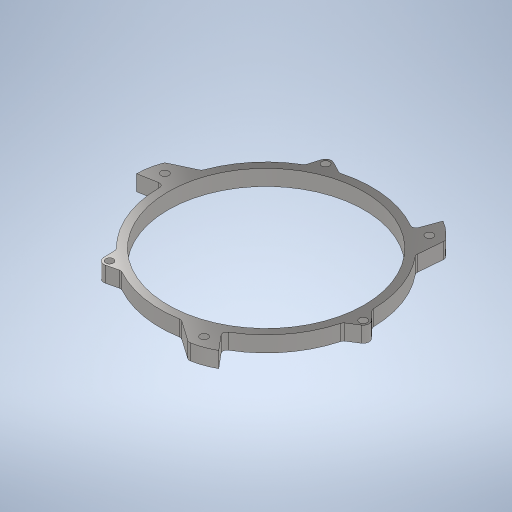
# Autodesk Inventor part: Blade V2
Saved by Autodesk Inventor 2023.2 (Build 272271000, 271)
## iProperties
Created: 2022-12-02
Part Number: Blade V2
Material: Stainless Steel
Document SubType Name: Modeling
Designer: Nathan Cai
Density: 8 g/cm^3
Appearance: Semi-Polished
Mass: 462.442 g
Surface Area: 248.364 cm^2
Volume: 57.8053 cm^3
Ring_ID: 6.250 in
ToothDepth: 0.750 in
RingWD: 0.250 in
Author: Nathan Cai
Autodesk Inventor part; units mm, degrees
ref_plane "YZ Plane" through (0, 0, 0) normal (1, 0, 0) x (0, 1, 0)
ref_plane "XZ Plane" through (0, 0, 0) normal (0, 1, 0) x (-1, 0, 0)
ref_plane "XY Plane" through (0, 0, 0) normal (0, 0, 1) x (1, 0, 0)
sketch "Sketch1" plane through (0, 0, 0) normal (0, 1, 0) x (-1, 0, 0)
  circle A0 centre (0, 0) radius 79.375
  circle A1 centre (0, 0) radius 85.725
  line L0 (0, 0) -> (104.775, 0) construction
  line L1 (104.775, 0) -> (85.6587, -3.3707)
  arc A2 (101.0679, -19.05) -> (104.775, 0) centre (53.975, 0) ccw
  arc A3 (91.7446, -23.4364) -> (97.7555, -7.6857) centre (53.975, 0) ccw construction
  line L2 (97.7555, -7.6857) -> (85.1505, -9.9083) construction
  circle A4 centre (93.5726, -11.6472) radius 3.175
  line L3 (101.0679, -19.05) -> (80.8223, -28.575)
  line L4 (93.5726, -11.6472) -> (-85.0685, 10.5887) construction
  circle A5 centre (-89.7946, 11.177) radius 4.7625
  circle A6 centre (-89.7946, 11.177) radius 3.175
  circle A7 centre (0, 0) radius 104.775 construction
  circle A8 centre (0, 0) radius 95.25 construction
  line L5 (-85.725, 0) -> (-93.2429, 7.8921)
  line L6 (-83.1092, 21.0152) -> (-92.3324, 15.2069)
  line L7 (42.8625, -74.24) -> (39.7867, -84.6968)
  line L8 (23.3549, -82.4823) -> (32.9966, -87.5657)
  circle A9 centre (35.2177, -83.3529) radius 4.7625
  circle A10 centre (35.2177, -83.3529) radius 3.175
  circle A11 centre (-36.6995, 86.8598) radius 3.175
  line L9 (-42.2218, 88.5016) -> (-33.9944, 78.6966) construction
  arc A12 (-25.5758, 91.1713) -> (-42.2218, 88.5016) centre (-26.9875, 46.7437) ccw construction
  line L10 (-34.0361, 97.0523) -> (-15.6645, 84.2817)
  line L11 (-52.3875, 90.7378) -> (-39.9102, 75.868)
  arc A13 (-34.0361, 97.0523) -> (-52.3875, 90.7378) centre (-26.9875, 46.7437) ccw
  line L12 (42.8625, 74.24) -> (53.4562, 76.8047)
  line L13 (59.7543, 61.467) -> (59.3358, 72.3587)
  circle A14 centre (54.5768, 72.1759) radius 4.7625
  circle A15 centre (54.5768, 72.1759) radius 3.175
  circle A16 centre (-56.8731, -75.2126) radius 3.175
  line L14 (-55.5338, -80.8159) -> (-51.1561, -68.7883) construction
  arc A17 (-66.1688, -67.7349) -> (-55.5338, -80.8159) centre (-26.9875, -46.7437) ccw construction
  line L15 (-67.0317, -78.0023) -> (-65.1578, -55.7067)
  line L16 (-52.3875, -90.7378) -> (-45.7485, -72.4973)
  arc A18 (-67.0317, -78.0023) -> (-52.3875, -90.7378) centre (-26.9875, -46.7437) ccw
  point P0 (85.725, 0)
  point P1 (33.3642, -78.9659)
  point P2 (-42.8625, 74.24)
  point P3 (51.7044, 68.3772)
  point P4 (-42.8625, -74.24)
  point P5 (-92.3324, 15.2069)
  point P6 (32.9966, -87.5657)
  point P7 (59.3358, 72.3587)
  dimension "d28" = 9.525
  dimension "d30" = 209.55
  dimension "Ring_ID" = 158.75
  dimension "RingWD" = 6.35
  dimension "ToothDepth" = 19.05
  dimension "d4" = 10
  dimension "d5" = 50.8
  dimension "d13" = 6.35
  dimension "d14" = 6.35
  dimension "d20" = 6.35
  dimension "d22" = 19.05
  dimension "d23" = 28.575
  dimension "d29" = 6.35
  dimension "d31" = 171.45
  dimension "d32" = 9.525
  dimension "d35" = 360
  constraints: 34 end point, 18 point on circle, 15 centre point, 7 coincident, 7 point on line, 2 symmetric about line, 2 tangent, 1 horizontal, 1 horizontal alignment, 1 line through centre, 96 other
  measures "Ring_ID" diameter of A0
  measures "RingWD" radial gap between concentric circles of A1 A0
  measures "ToothDepth" distance of A1.start L0.end
  measures "d4" angle of L0 L1
  measures "d5" radius of A2
  measures "d13" radial gap between concentric circles of A2 A3
  measures "d14" distance between parallel lines of L1 L2
  measures "d20" diameter of A4
  measures "d22" vertical distance of L3.start L0.end
  measures "d23" distance from line of L0 L3.end
  measures "d29" diameter of A6
  measures "d31" diameter of A1
extrude "Extrusion1" add sketch "Sketch1" along normal blind 12.7
fillet "Fillet1" radius 3.175 15 edges at (-85.6587, 6.35, -3.3707) (-101.0679, 6.35, -19.05) (-80.8223, 6.35, -28.575) (-42.8625, 6.35, -74.24) (-23.3549, 6.35, -82.4823) (45.7485, 6.35, -72.4973) (65.1578, 6.35, -55.7067) (85.725, 6.35, 0) (83.1092, 6.35, 21.0152) (39.9102, 6.35, 75.868) (34.0361, 6.35, 97.0523) (15.6645, 6.35, 84.2817) (-42.8625, 6.35, 74.24) (-59.7543, 6.35, 61.467) (67.0317, 6.35, -78.0023)
body "Solid1"
